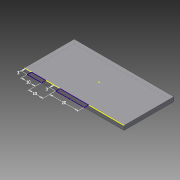
# Autodesk Inventor part: Lower bottom
Saved by Autodesk Inventor 2015 (Build 190159000, 159)
## iProperties
Created: 2014-11-12
Part Number: Lower bottom
Material: Generic
Document SubType Name: Modeling
Designer: karl
Density: 1 g/cm^3
Appearance: Default
Author: karl
Autodesk Inventor part; units mm, degrees
ref_plane "YZ Plane" through (0, 0, 0) normal (1, 0, 0) x (0, 1, 0)
ref_plane "XZ Plane" through (0, 0, 0) normal (0, 1, 0) x (-1, 0, 0)
ref_plane "XY Plane" through (0, 0, 0) normal (0, 0, 1) x (1, 0, 0)
sketch "Sketch1" plane through (0, 0, 0) normal (0, 0, 1) x (1, 0, 0)
  line L0 (57, -17.5) -> (-57, -17.5)
  line L1 (-57, -17.5) -> (-57, 17.5)
  line L2 (-57, 17.5) -> (57, 17.5)
  line L3 (57, 17.5) -> (57, -17.5)
  line L4 (57, -17.5) -> (-57, 17.5) construction
  line L5 (-57, -17.5) -> (57, 17.5) construction
  point P0 (0, 0)
  dimension "d0" = 114
  dimension "d1" = 35
  constraints: 12 end point, 2 midpoint, 2 parallel, 1 horizontal, 1 perpendicular
  measures "d0" distance of L1.end L2.end
  measures "d1" distance of L0.end L1.end
extrude "Extrusion1" add sketch "Sketch1" along normal blind 3
sketch "Sketch2" plane through (0, 0, 3) normal (0, 0, 1) x (1, 0, 0)
  line L0 (-57, -17.5) -> (57, -17.5) projected
  line L1 (10, -17.5) -> (-10, -17.5)
  line L2 (-10, -17.5) -> (-10, -20.5)
  line L3 (-10, -20.5) -> (10, -20.5)
  line L4 (10, -20.5) -> (10, -17.5)
  line L5 (-20, -17.5) -> (-25, -17.5)
  line L6 (-25, -17.5) -> (-25, -20.5)
  line L7 (-25, -20.5) -> (-20, -20.5)
  line L8 (-20, -20.5) -> (-20, -17.5)
  line L9 (20, -17.5) -> (25, -17.5)
  line L10 (25, -17.5) -> (25, -20.5)
  line L11 (25, -20.5) -> (20, -20.5)
  line L12 (20, -20.5) -> (20, -17.5)
  point P0 (0, 0)
  point P1 (0, -20.5)
  dimension "d4" = 20
  dimension "d5" = 3
  dimension "d6" = 5
  dimension "d7" = 3
  dimension "d8" = 10
  dimension "d9" = 5
  dimension "d10" = 3
  dimension "d11" = 10
  constraints: 24 end point, 6 parallel, 3 horizontal, 3 perpendicular, 3 point on line, 1 midpoint, 1 vertical alignment
  measures "d4" distance of L3.end L2.end
  measures "d5" distance of L2.end L1.end
  measures "d6" distance of L7.end L6.end
  measures "d7" distance of L6.end L5.end
  measures "d8" distance between parallel lines of L2 L8
  measures "d9" distance of L10.end L11.end
  measures "d10" distance of L9.end L10.end
  measures "d11" distance between parallel lines of L12 L4
extrude "Extrusion2" add sketch "Sketch2" against normal blind 3
sketch "Sketch3" plane through (0, 0, 0) normal (0, 0, -1) x (-1, 0, 0)
  line L0 (57, -17.5) -> (25, -17.5) projected
  line L1 (38, -17.5) -> (35, -17.5)
  line L2 (35, -17.5) -> (35, 2.5)
  line L3 (35, 2.5) -> (38, 2.5)
  line L4 (38, 2.5) -> (38, -17.5)
  line L5 (-57, 17.5) -> (57, 17.5) projected
  point P0 (0, 0)
  dimension "d14" = 3
  dimension "d15" = 15
  dimension "d16" = 35
  constraints: 8 end point, 2 parallel, 1 horizontal, 1 perpendicular, 1 point on line
  measures "d14" distance of L2.end L3.end
  measures "d15" distance between parallel lines of L5 L3
  measures "d16" distance from line of point (0, 0) L2
extrude "Extrusion3" cut sketch "Sketch3" against normal blind 3
sketch "Sketch4" plane through (0, 0, 0) normal (0, 0, -1) x (-1, 0, 0)
  line L0 (38, -17.5) -> (57, -17.5) projected
  line L1 (42, -17.5) -> (52, -17.5)
  line L2 (52, -17.5) -> (52, -20.5)
  line L3 (52, -20.5) -> (42, -20.5)
  line L4 (42, -20.5) -> (42, -17.5)
  line L5 (25, -20.5) -> (25, -17.5) projected
  point P0 (0, 0)
  dimension "d19" = 10
  dimension "d20" = 3
  dimension "d21" = 17
  constraints: 8 end point, 2 parallel, 1 horizontal, 1 perpendicular, 1 point on line
  measures "d19" distance of L2.end L3.end
  measures "d20" distance of L1.end L2.end
  measures "d21" distance between parallel lines of L5 L4
extrude "Extrusion4" add sketch "Sketch4" against normal blind 3
sketch "Sketch5" plane through (0, 0, 0) normal (0, 0, -1) x (-1, 0, 0)
  line L0 (57, 17.5) -> (57, -17.5) projected
  line L1 (57, -10) -> (60, -10)
  line L2 (60, -10) -> (60, 10)
  line L3 (60, 10) -> (57, 10)
  line L4 (57, 10) -> (57, -10)
  line L5 (52, -17.5) -> (57, -17.5) projected
  point P0 (0, 0)
  dimension "d24" = 3
  dimension "d25" = 20
  dimension "d26" = 7.5
  constraints: 8 end point, 2 parallel, 1 horizontal, 1 perpendicular, 1 point on line
  measures "d24" distance of L3.end L2.end
  measures "d25" distance of L2.end L1.end
  measures "d26" distance between parallel lines of L5 L1
extrude "Extrusion5" add sketch "Sketch5" against normal blind 3
mirror "Mirror1" about plane through (0, 0, 0) normal (1, 0, 0) of "Extrusion5", "Extrusion4", "Extrusion3"
sketch "Sketch6" plane through (0, 0, 3) normal (0, 0, 1) x (1, 0, 0)
  line L0 (-57, 17.5) -> (57, 17.5) projected
  line L1 (52.5, 17.5) -> (42.5, 17.5)
  line L2 (42.5, 17.5) -> (42.5, 20.5)
  line L3 (42.5, 20.5) -> (52.5, 20.5)
  line L4 (52.5, 20.5) -> (52.5, 17.5)
  line L5 (25, 17.5) -> (5, 17.5)
  line L6 (5, 17.5) -> (5, 20.5)
  line L7 (5, 20.5) -> (25, 20.5)
  line L8 (25, 20.5) -> (25, 17.5)
  point P0 (0, 0)
  dimension "d29" = 10
  dimension "d30" = 3
  dimension "d31" = 20
  dimension "d32" = 3
  dimension "d33" = 17.5
  dimension "d34" = 5
  constraints: 16 end point, 4 parallel, 2 horizontal, 2 perpendicular, 2 point on line
  measures "d29" distance of L2.end L3.end
  measures "d30" distance of L1.end L2.end
  measures "d31" distance of L6.end L7.end
  measures "d32" distance of L5.end L6.end
  measures "d33" distance between parallel lines of L2 L8
  measures "d34" distance from line of point (0, 0) L6
extrude "Extrusion6" add sketch "Sketch6" against normal blind 3
sketch "Sketch7" plane through (0, 0, 3) normal (0, 0, 1) x (1, 0, 0)
  line L0 (25, 9) -> (25, -9) construction
  line L1 (20, 9) -> (20, -9)
  line L2 (30, -9) -> (30, 9)
  arc A0 (30, 9) -> (20, 9) centre (25, 9) ccw
  arc A1 (20, -9) -> (30, -9) centre (25, -9) ccw
  point P0 (0, 0)
  point P1 (25, 0)
  dimension "d37" = 18
  dimension "d38" = 10
  dimension "d39" = 25
  constraints: 8 end point, 4 point on circle, 4 tangent, 2 centre point, 1 horizontal alignment, 1 midpoint, 1 parallel, 1 vertical
  measures "d37" distance of L0.start L0.end
  measures "d38" diameter of A1
  measures "d39" distance from line of point (0, 0) L0
extrude "Extrusion7" cut sketch "Sketch7" against normal blind 3
sketch "Sketch8" plane through (0, 0, 3) normal (0, 0, 1) x (1, 0, 0)
  line L0 (12.5, 12) -> (-12.5, 12) construction
  line L1 (12.5, 13.5) -> (-12.5, 13.5)
  line L2 (-12.5, 10.5) -> (12.5, 10.5)
  arc A0 (12.5, 10.5) -> (12.5, 13.5) centre (12.5, 12) ccw
  arc A1 (-12.5, 13.5) -> (-12.5, 10.5) centre (-12.5, 12) ccw
  line L3 (-12.5, 6) -> (12.5, 6) construction
  line L4 (-12.5, 4.5) -> (12.5, 4.5)
  line L5 (12.5, 7.5) -> (-12.5, 7.5)
  arc A2 (-12.5, 7.5) -> (-12.5, 4.5) centre (-12.5, 6) ccw
  arc A3 (12.5, 4.5) -> (12.5, 7.5) centre (12.5, 6) ccw
  line L6 (-12.5, -6) -> (12.5, -6) construction
  line L7 (-12.5, -7.5) -> (12.5, -7.5)
  line L8 (12.5, -4.5) -> (-12.5, -4.5)
  arc A4 (-12.5, -4.5) -> (-12.5, -7.5) centre (-12.5, -6) ccw
  arc A5 (12.5, -7.5) -> (12.5, -4.5) centre (12.5, -6) ccw
  line L9 (-12.5, -12) -> (12.5, -12) construction
  line L10 (-12.5, -13.5) -> (12.5, -13.5)
  line L11 (12.5, -10.5) -> (-12.5, -10.5)
  arc A6 (-12.5, -10.5) -> (-12.5, -13.5) centre (-12.5, -12) ccw
  arc A7 (12.5, -13.5) -> (12.5, -10.5) centre (12.5, -12) ccw
  line L12 (-12.5, 0) -> (12.5, 0) construction
  line L13 (-12.5, -1.5) -> (12.5, -1.5)
  line L14 (12.5, 1.5) -> (-12.5, 1.5)
  arc A8 (-12.5, 1.5) -> (-12.5, -1.5) centre (-12.5, 0) ccw
  arc A9 (12.5, -1.5) -> (12.5, 1.5) centre (12.5, 0) ccw
  point P0 (0, 0)
  point P1 (0, 12)
  point P2 (0, 6)
  point P3 (0, -6)
  point P4 (0, -12)
  point P5 (0, 0)
  dimension "d42" = 3
  dimension "d43" = 12
  dimension "d44" = 3
  dimension "d45" = 3
  dimension "d46" = 3
  dimension "d47" = 12
  dimension "d48" = 6
  dimension "d49" = 6
  dimension "d50" = 3
  dimension "d51" = 25
  constraints: 40 end point, 20 point on circle, 20 tangent, 10 centre point, 8 vertical alignment, 7 parallel, 5 midpoint, 3 horizontal, 1 coincident
  measures "d42" diameter of A1
  measures "d43" distance from line of point (0, 0) L0
  measures "d44" diameter of A3
  measures "d45" diameter of A5
  measures "d46" diameter of A7
  measures "d47" distance from line of L9 point (0, 0)
  measures "d48" distance from line of point (0, 0) L6
  measures "d49" distance from line of point (0, 0) L3
  measures "d50" diameter of A9
  measures "d51" distance of L0.start L0.end
extrude "Extrusion8" cut sketch "Sketch8" against normal blind 3
mirror "Mirror2" about plane through (0, 0, 0) normal (1, 0, 0) of "Extrusion6", "Extrusion7"
equation "\"d11\" = d8"
equation "\"d47\" = d43"
equation "\"d49\" = d48"
body "Solid1"
